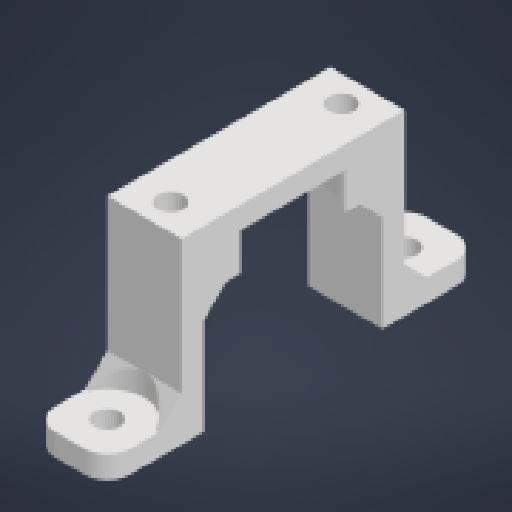
# Autodesk Inventor part: Small Gear Bracket
Saved by Autodesk Inventor 2023 (Build 270158000, 158)
## iProperties
Created: 2022-11-20
Part Number: Small Gear Bracket
Material: Generic
Document SubType Name: Modeling
Designer: Izack Waczko
Density: 1 g/cm^3
Appearance: Default
Author: Izack Waczko
Autodesk Inventor part; units mm, degrees
ref_plane "YZ Plane" through (0, 0, 0) normal (1, 0, 0) x (0, 1, 0)
ref_plane "XZ Plane" through (0, 0, 0) normal (0, 1, 0) x (-1, 0, 0)
ref_plane "XY Plane" through (0, 0, 0) normal (0, 0, 1) x (1, 0, 0)
sketch "Sketch1" plane through (0, 0, 0) normal (0, 1, 0) x (-1, 0, 0)
  line L0 (0, 0) -> (0, -40) construction
  circle A0 centre (0, 0) radius 1.7
  circle A1 centre (0, -40) radius 1.7
  line L1 (-5, -5) -> (5, -5)
  line L2 (5, -5) -> (5, 2)
  line L3 (2, 5) -> (-2, 5)
  line L4 (-5, 2) -> (-5, -5)
  line L5 (-5, -5) -> (5, 5) construction
  line L6 (5, -5) -> (-5, 5) construction
  line L7 (-5, -35) -> (5, -35)
  line L8 (5, -35) -> (5, -42)
  line L9 (2, -45) -> (-2, -45)
  line L10 (-5, -42) -> (-5, -35)
  line L11 (-5, -35) -> (5, -45) construction
  line L12 (5, -35) -> (-5, -45) construction
  arc A2 (5, 2) -> (2, 5) centre (2, 2) ccw
  arc A3 (-2, 5) -> (-5, 2) centre (-2, 2) ccw
  arc A4 (-5, -42) -> (-2, -45) centre (-2, -42) ccw
  arc A5 (2, -45) -> (5, -42) centre (2, -42) ccw
  line L13 (5, -5) -> (5, -35)
  line L14 (-5, -5) -> (-5, -35)
  line L15 (5, -5) -> (-5, -5)
  line L16 (-5, -5) -> (-5, -8)
  line L17 (-5, -8) -> (5, -8)
  line L18 (5, -8) -> (5, -5)
  line L19 (5, -35) -> (-5, -35)
  line L20 (-5, -35) -> (-5, -32)
  line L21 (-5, -32) -> (5, -32)
  line L22 (5, -32) -> (5, -35)
  dimension "d0" = 40
  dimension "d1" = 3.4
  dimension "d2" = 3.4
  dimension "d3" = 10
  dimension "d4" = 10
  dimension "d5" = 10
  dimension "d6" = 10
  dimension "d7" = 3
  dimension "d10" = 3
  dimension "d11" = 3
  constraints: 46 end point, 10 point on line, 8 parallel, 8 point on circle, 8 tangent, 6 centre point, 4 horizontal, 4 midpoint, 4 perpendicular, 3 equal radius, 2 coincident, 1 vertical
  measures "d0" distance of L0.start L0.end
  measures "d1" diameter of A0
  measures "d2" diameter of A1
  measures "d3" distance of L6.end L5.end
  measures "d4" distance of L5.end L1.end
  measures "d5" distance of L11.end L12.end
  measures "d6" distance of L7.end L11.end
  measures "d7" radius of A2
  measures "d10" distance of L16.end L15.end
  measures "d11" distance of L19.end L20.end
extrude "Extrusion1" add sketch "Sketch1" along normal blind 3 contours L4 A3 L3 A2 L2 L1 | L7 L8 A5 L9 A4 L10
extrude "Extrusion2" add sketch "Sketch1" along normal blind 16 contours L1 L13 L17 L14 | L21 L13 L7 L14
sketch "Sketch2" plane through (0, 16, 0) normal (0, 1, 0) x (1, 0, 0)
  line L0 (0, 7.9504) -> (0, 32) construction
  line L1 (-5, 32) -> (5, 32) projected
  circle A0 centre (0, 19.9752) radius 8.65
  line L2 (-5, 5) -> (5, 5)
  line L3 (5, 5) -> (5, 12.9167)
  line L4 (5, 12.9167) -> (-5, 12.9167)
  line L5 (-5, 12.9167) -> (-5, 5)
  line L6 (-5, 42) -> (-5, 35) projected
  line L7 (-5, 35) -> (5, 35)
  line L8 (5, 35) -> (5, 27.0337)
  line L9 (5, 27.0337) -> (-5, 27.0337)
  line L10 (-5, 27.0337) -> (-5, 35)
  point P0 (0, 0)
  dimension "d14" = 17.3
  constraints: 18 end point, 4 parallel, 2 horizontal, 2 midpoint, 2 perpendicular, 2 point on circle, 1 centre point, 1 point on line
  measures "d14" diameter of A0
extrude "Extrusion3" add sketch "Sketch2" along normal blind 5 contours L10 L7 L8 L1 | L1 L8 A0 L10 | A0 L3 L2 L5
sketch "Sketch3" plane through (0, 21, 0) normal (0, 1, 0) x (1, 0, 0)
  line L0 (-5, 5) -> (-5, -2) projected
  line L1 (5, 35) -> (5, 42) projected
  line L2 (-5, 5) -> (5, 5)
  line L3 (5, 5) -> (5, 35)
  line L4 (5, 35) -> (-5, 35)
  line L5 (-5, 35) -> (-5, 5)
  point P0 (0, 0)
  constraints: 8 end point, 2 parallel, 1 horizontal, 1 perpendicular
extrude "Extrusion4" add sketch "Sketch3" along normal blind 3
chamfer "Chamfer2" distance 3 angle 45 4 edges at (0, 16, -8) (0, 16, -32) (0, 3, -35) (0, 3, -5)
sketch "Sketch5" plane through (0, 24, 0) normal (0, 1, 0) x (1, 0, 0)
  line L0 (5, 35) -> (-5, 35) construction
  line L1 (0, 35) -> (0, 5) construction
  line L2 (-5, 5) -> (5, 5) construction
  circle A0 centre (0, 31.5) radius 1.7
  circle A1 centre (0, 8.5) radius 1.7
  point P0 (0, 0)
  dimension "d29" = 3.4
  dimension "d30" = 3.4
  dimension "d31" = 3.5
  dimension "d32" = 3.5
  constraints: 2 centre point, 2 end point, 2 midpoint, 2 point on line
  measures "d29" diameter of A0
  measures "d30" diameter of A1
  measures "d31" distance from line of L0 A0.centre
  measures "d32" distance from line of L2 A1.centre
extrude "Extrusion6" cut sketch "Sketch5" against normal blind 8
sketch "Sketch6" plane through (0, 3, 0) normal (0, 1, 0) x (1, 0, 0)
  circle A0 centre (0, 0) radius 5
  circle A1 centre (0, 40) radius 1.7 projected
  circle A2 centre (0, 40) radius 5
  dimension "d35" = 10
  dimension "d36" = 10
  constraints: 2 centre point, 2 coincident
  measures "d35" diameter of A0
  measures "d36" diameter of A2
extrude "Extrusion7" cut sketch "Sketch6" along normal blind 10
body "Solid1"
